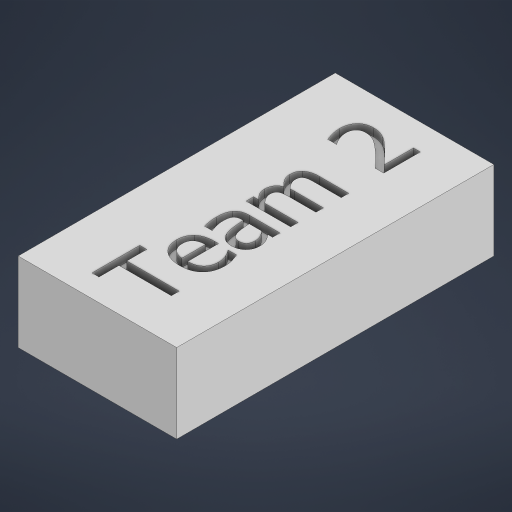
# Autodesk Inventor part: Project1Part
Saved by Autodesk Inventor 2023 (Build 270158000, 158)
## iProperties
Created: 2023-01-31
Part Number: Project1Part
Material: Generic
Document SubType Name: Modeling
Designer: Aidan Gowe
Density: 1 g/cm^3
Appearance: Default
Author: Aidan Gowe
Autodesk Inventor part; units mm, degrees
note: some values were not read from the file. Chosen so that the rebuilt part matches the saved one: direction of "Emboss1".
ref_plane "YZ Plane" through (0, 0, 0) normal (1, 0, 0) x (0, 1, 0)
ref_plane "XZ Plane" through (0, 0, 0) normal (0, 1, 0) x (-1, 0, 0)
ref_plane "XY Plane" through (0, 0, 0) normal (0, 0, 1) x (1, 0, 0)
sketch "Sketch1" plane through (0, 0, 0) normal (0, 1, 0) x (-1, 0, 0)
  line L0 (0, -50.8) -> (25.4, -50.8)
  line L1 (25.4, -50.8) -> (25.4, 50.8)
  line L2 (25.4, 50.8) -> (-25.4, 50.8)
  line L3 (-25.4, 50.8) -> (-25.4, -50.8)
  line L4 (-25.4, -50.8) -> (0, -50.8)
  point P0 (0, 0)
  dimension "d1" = 25.4
  dimension "d2" = 101.6
  dimension "d3" = 50.8
  dimension "d4" = 101.6
  constraints: 10 end point, 2 perpendicular, 1 horizontal, 1 point on line
  measures "d1" distance of L0.start L0.end
  measures "d2" distance of L0.end L1.end
  measures "d3" distance of L1.end L2.end
  measures "d4" distance of L2.end L3.end
extrude "Extrusion1" add sketch "Sketch1" along normal blind 25.4
sketch "Sketch2" plane through (0, 25.4, 0) normal (0, 1, 0) x (1, 0, 0)
  line L0 (-25.4, 50.8) -> (-25.4, -50.8) projected
  line L1 (-25.4, -50.8) -> (-25.4, 50.8)
  line L2 (25.4, 50.8) -> (-25.4, 50.8) projected
  line L3 (-25.4, 50.8) -> (25.4, 50.8)
  line L4 (25.4, -50.8) -> (25.4, 50.8) projected
  line L5 (25.4, 50.8) -> (25.4, -50.8)
  line L6 (-25.4, -50.8) -> (25.4, -50.8) projected
  line L7 (25.4, -50.8) -> (-25.4, -50.8)
  line L8 (10.16, -37.2818) -> (-6.6361, -37.2818)
  line L9 (-6.6361, -37.2818) -> (-6.6361, -43.673)
  line L10 (-6.6361, -43.673) -> (-8.89, -43.673)
  line L11 (-8.89, -43.673) -> (-8.89, -28.3589)
  line L12 (-8.89, -28.3589) -> (-6.6361, -28.3589)
  line L13 (-6.6361, -28.3589) -> (-6.6361, -34.75)
  line L14 (-6.6361, -34.75) -> (10.16, -34.75)
  line L15 (10.16, -34.75) -> (10.16, -37.2818)
  spline S0 degree 2 poles (10.4842, -20.3931) (10.4842, -23.8202) (6.6402, -27.587) (3.0896, -27.587) knots 0 0 0 1 2 2 2
  spline S1 degree 2 poles (3.0896, -27.587) (-0.3993, -27.587) (-4.5366, -23.9283) (-4.5366, -20.9797) knots 0 0 0 1 2 2 2
  spline S2 degree 2 poles (-4.5366, -20.9797) (-4.5366, -19.6521) (-3.7647, -17.5989) (-2.9465, -16.8424) knots 0 0 0 1 2 2 2
  spline S3 degree 2 poles (-2.9465, -16.8424) (-2.1283, -16.0705) (0.2336, -15.2524) (1.9472, -15.2524) knots 0 0 0 1 2 2 2
  line L16 (1.9472, -15.2524) -> (3.2594, -15.2524)
  line L17 (3.2594, -15.2524) -> (3.2594, -25.1479)
  spline S4 degree 2 poles (3.2594, -25.1479) (5.7448, -25.1479) (8.3847, -22.647) (8.3847, -20.4239) knots 0 0 0 1 2 2 2
  spline S5 degree 2 poles (8.3847, -20.4239) (8.3847, -19.6366) (8.0296, -18.1083) (7.7517, -17.4908) knots 0 0 0 1 2 2 2
  spline S6 degree 2 poles (7.7517, -17.4908) (7.443, -16.8424) (6.9027, -15.947) (6.6557, -15.6537) knots 0 0 0 1 2 2 2
  line L18 (6.6557, -15.6537) -> (6.6557, -15.5148)
  line L19 (6.6557, -15.5148) -> (9.2801, -15.5148)
  spline S7 degree 2 poles (9.2801, -15.5148) (9.4499, -15.9316) (9.9439, -17.1975) (10.0828, -17.6915) knots 0 0 0 1 2 2 2
  spline S8 degree 2 poles (10.0828, -17.6915) (10.2835, -18.3862) (10.4842, -19.5286) (10.4842, -20.3931) knots 0 0 0 1 2 2 2
  spline S9 degree 2 poles (1.4223, -17.5989) (0.4497, -17.6297) (-0.9705, -18.0311) (-1.4491, -18.4171) knots 0 0 0 1 2 2 2
  spline S10 degree 2 poles (-1.4491, -18.4171) (-1.9894, -18.8339) (-2.5606, -20.1461) (-2.5606, -21.1186) knots 0 0 0 1 2 2 2
  spline S11 degree 2 poles (-2.5606, -21.1186) (-2.5606, -22.0758) (-1.9894, -23.4188) (-1.4336, -23.9746) knots 0 0 0 1 2 2 2
  spline S12 degree 2 poles (-1.4336, -23.9746) (-0.8624, -24.5149) (0.5115, -25.0707) (1.4223, -25.1479) knots 0 0 0 1 2 2 2
  line L20 (1.4223, -25.1479) -> (1.4223, -17.5989)
  spline S13 degree 2 poles (8.6471, -4.8474) (8.8632, -5.1407) (9.6351, -6.1287) (9.8667, -6.5919) knots 0 0 0 1 2 2 2
  spline S14 degree 2 poles (9.8667, -6.5919) (10.2063, -7.2248) (10.5614, -8.4135) (10.5614, -9.4941) knots 0 0 0 1 2 2 2
  spline S15 degree 2 poles (10.5614, -9.4941) (10.5614, -10.3741) (9.8976, -11.9641) (9.2955, -12.5662) knots 0 0 0 1 2 2 2
  spline S16 degree 2 poles (9.2955, -12.5662) (8.7089, -13.1374) (6.9799, -13.8321) (6.0227, -13.8321) knots 0 0 0 1 2 2 2
  spline S17 degree 2 poles (6.0227, -13.8321) (4.5407, -13.8321) (2.4412, -12.5816) (1.8391, -11.2231) knots 0 0 0 1 2 2 2
  spline S18 degree 2 poles (1.8391, -11.2231) (1.2834, -10.019) (0.8666, -6.7462) (0.7585, -4.8474) knots 0 0 0 1 2 2 2
  line L21 (0.7585, -4.8474) -> (0.2954, -4.8474)
  spline S19 degree 2 poles (0.2954, -4.8474) (-0.5383, -4.8474) (-1.5726, -5.3568) (-1.8659, -5.82) knots 0 0 0 1 2 2 2
  spline S20 degree 2 poles (-1.8659, -5.82) (-2.1592, -6.2831) (-2.3445, -7.6107) (-2.3445, -8.3209) knots 0 0 0 1 2 2 2
  spline S21 degree 2 poles (-2.3445, -8.3209) (-2.3445, -9.1545) (-1.8505, -11.4084) (-1.3719, -12.5353) knots 0 0 0 1 2 2 2
  line L22 (-1.3719, -12.5353) -> (-1.3719, -12.6743)
  line L23 (-1.3719, -12.6743) -> (-3.8265, -12.6743)
  spline S22 degree 2 poles (-3.8265, -12.6743) (-4.0117, -12.0105) (-4.4748, -9.525) (-4.4748, -8.3054) knots 0 0 0 1 2 2 2
  spline S23 degree 2 poles (-4.4748, -8.3054) (-4.4748, -6.8234) (-4.0117, -4.8011) (-3.4097, -3.9983) knots 0 0 0 1 2 2 2
  spline S24 degree 2 poles (-3.4097, -3.9983) (-2.823, -3.211) (-0.9551, -2.4391) (0.388, -2.4391) knots 0 0 0 1 2 2 2
  line L24 (0.388, -2.4391) -> (10.16, -2.4391)
  line L25 (10.16, -2.4391) -> (10.16, -4.8474)
  line L26 (10.16, -4.8474) -> (8.6471, -4.8474)
  line L27 (6.6402, -4.8474) -> (2.6728, -4.8474)
  spline S25 degree 2 poles (2.6728, -4.8474) (2.75, -5.7119) (3.0124, -8.3209) (3.2594, -9.1391) knots 0 0 0 1 2 2 2
  spline S26 degree 2 poles (3.2594, -9.1391) (3.5527, -10.0962) (4.7723, -11.3466) (5.8529, -11.3466) knots 0 0 0 1 2 2 2
  spline S27 degree 2 poles (5.8529, -11.3466) (7.0879, -11.3466) (8.3384, -9.9573) (8.3384, -8.6296) knots 0 0 0 1 2 2 2
  spline S28 degree 2 poles (8.3384, -8.6296) (8.3384, -7.5027) (7.3658, -5.6502) (6.6402, -4.8474) knots 0 0 0 1 2 2 2
  line L28 (10.16, 17.1512) -> (1.8854, 17.1512)
  spline S29 degree 2 poles (1.8854, 17.1512) (0.8974, 17.1512) (-0.7853, 16.9968) (-1.2484, 16.7498) knots 0 0 0 1 2 2 2
  spline S30 degree 2 poles (-1.2484, 16.7498) (-1.7578, 16.5028) (-2.2518, 15.5611) (-2.2518, 14.7429) knots 0 0 0 1 2 2 2
  spline S31 degree 2 poles (-2.2518, 14.7429) (-2.2518, 14.0019) (-1.341, 12.3038) (-0.4765, 11.4084) knots 0 0 0 1 2 2 2
  spline S32 degree 2 poles (-0.4765, 11.4084) (-0.2604, 11.4238) (0.3417, 11.4547) (0.7431, 11.4547) knots 0 0 0 1 2 2 2
  line L29 (0.7431, 11.4547) -> (10.16, 11.4547)
  line L30 (10.16, 11.4547) -> (10.16, 9.0464)
  line L31 (10.16, 9.0464) -> (1.8854, 9.0464)
  spline S33 degree 2 poles (1.8854, 9.0464) (0.8974, 9.0464) (-0.7853, 8.8921) (-1.2484, 8.6451) knots 0 0 0 1 2 2 2
  spline S34 degree 2 poles (-1.2484, 8.6451) (-1.7578, 8.3981) (-2.2518, 7.4564) (-2.2518, 6.6382) knots 0 0 0 1 2 2 2
  spline S35 degree 2 poles (-2.2518, 6.6382) (-2.2518, 5.8663) (-1.2793, 4.1527) (-0.5228, 3.35) knots 0 0 0 1 2 2 2
  line L32 (-0.5228, 3.35) -> (10.16, 3.35)
  line L33 (10.16, 3.35) -> (10.16, 0.9417)
  line L34 (10.16, 0.9417) -> (-4.1352, 0.9417)
  line L35 (-4.1352, 0.9417) -> (-4.1352, 3.35)
  line L36 (-4.1352, 3.35) -> (-2.5606, 3.35)
  spline S36 degree 2 poles (-2.5606, 3.35) (-3.5023, 4.2917) (-4.5366, 6.1442) (-4.5366, 7.2557) knots 0 0 0 1 2 2 2
  spline S37 degree 2 poles (-4.5366, 7.2557) (-4.5366, 8.5216) (-3.3788, 10.4821) (-2.0666, 10.9916) knots 0 0 0 1 2 2 2
  spline S38 degree 2 poles (-2.0666, 10.9916) (-3.2862, 12.0876) (-4.5366, 14.1563) (-4.5366, 15.3604) knots 0 0 0 1 2 2 2
  spline S39 degree 2 poles (-4.5366, 15.3604) (-4.5366, 16.2867) (-3.9654, 17.7996) (-3.317, 18.3553) knots 0 0 0 1 2 2 2
  spline S40 degree 2 poles (-3.317, 18.3553) (-2.6686, 18.9265) (-0.7235, 19.5594) (0.7431, 19.5594) knots 0 0 0 1 2 2 2
  line L37 (0.7431, 19.5594) -> (10.16, 19.5594)
  line L38 (10.16, 19.5594) -> (10.16, 17.1512)
  line L39 (10.16, 42.5152) -> (10.16, 30.7671)
  line L40 (10.16, 30.7671) -> (7.4584, 30.7671)
  spline S41 degree 2 poles (7.4584, 30.7671) (6.2697, 32.033) (4.0621, 34.2869) (2.8735, 35.3675) knots 0 0 0 1 2 2 2
  spline S42 degree 2 poles (2.8735, 35.3675) (0.4806, 37.5442) (-2.3908, 39.1343) (-3.9191, 39.1343) knots 0 0 0 1 2 2 2
  spline S43 degree 2 poles (-3.9191, 39.1343) (-4.7218, 39.1343) (-5.926, 38.6403) (-6.3119, 38.1926) knots 0 0 0 1 2 2 2
  spline S44 degree 2 poles (-6.3119, 38.1926) (-6.6979, 37.7449) (-7.0838, 36.5717) (-7.0838, 35.8615) knots 0 0 0 1 2 2 2
  spline S45 degree 2 poles (-7.0838, 35.8615) (-7.0838, 35.1823) (-6.7442, 33.7929) (-6.4817, 33.16) knots 0 0 0 1 2 2 2
  spline S46 degree 2 poles (-6.4817, 33.16) (-6.2656, 32.6196) (-5.6481, 31.6162) (-5.432, 31.3075) knots 0 0 0 1 2 2 2
  line L41 (-5.432, 31.3075) -> (-5.432, 31.1685)
  line L42 (-5.432, 31.1685) -> (-8.149, 31.1685)
  spline S47 degree 2 poles (-8.149, 31.1685) (-8.5349, 31.9558) (-9.2914, 34.7809) (-9.2914, 36.0468) knots 0 0 0 1 2 2 2
  spline S48 degree 2 poles (-9.2914, 36.0468) (-9.2914, 38.7175) (-6.4663, 41.7278) (-4.058, 41.7278) knots 0 0 0 1 2 2 2
  spline S49 degree 2 poles (-4.058, 41.7278) (-2.9311, 41.7278) (-1.0477, 41.203) (-0.2449, 40.7398) knots 0 0 0 1 2 2 2
  spline S50 degree 2 poles (-0.2449, 40.7398) (0.5887, 40.2767) (2.2251, 38.9336) (3.0124, 38.1926) knots 0 0 0 1 2 2 2
  spline S51 degree 2 poles (3.0124, 38.1926) (4.3246, 36.9885) (7.1342, 34.0399) (7.9524, 33.16) knots 0 0 0 1 2 2 2
  line L43 (7.9524, 33.16) -> (7.9524, 42.5152)
  line L44 (7.9524, 42.5152) -> (10.16, 42.5152)
  point P0 (0, 0)
  constraints: 8 end point, 2 collinear, 2 vertical, 1 perpendicular
emboss "Emboss1" sketch "Sketch2" operation cut depth 2.54 direction (0, -1, 0) contours L8 L9 L10 L11 L12 L13 L14 L15 | S0 S1 S2 S3 L16 L17 S4 S5 S6 L18 L19 S7 S8 | S13 S14 S15 S16 S17 S18 L21 S19 S20 S21 L22 L23 S22 S23 S24 L24 L25 L26 | L28 S29 S30 S31 S32 L29 L30 L31 S33 S34 S35 L32 L33 L34 L35 L36 S36 S37 S38 S39 S40 L37 L38 | L39 L40 S41 S42 S43 S44 S45 S46 L41 L42 S47 S48 S49 S50 S51 L43 L44
body "Solid1"
